Autodesk Fusion 360 part; units mm, degrees
(part 2 of 2)
  constraint perpendicular L102 L652
  constraint perpendicular L102 L126
  constraint perpendicular L121 L652
  constraint perpendicular L117 L121
  constraint perpendicular L572 L652
  constraint perpendicular L47 L572
  constraint perpendicular L83 L132
  constraint perpendicular L185 L219
  constraint perpendicular L70 L132
  constraint perpendicular L55 L185
  constraint perpendicular L132 L662
  constraint perpendicular L185 L660
  constraint perpendicular L132 L188
  constraint perpendicular L183 L185
  constraint perpendicular L16 L132
  constraint perpendicular L185 L686
  constraint perpendicular L132 L681
  constraint perpendicular L185 L684
  constraint perpendicular L132 L676
  constraint perpendicular L185 L690
  constraint perpendicular L685 L690
  constraint perpendicular L685 L689
  constraint perpendicular L690 L695
  constraint perpendicular L693 L695
  constraint perpendicular L690 L691
  constraint perpendicular L691 L703
  constraint perpendicular L690 L694
  constraint perpendicular L679 L694
  constraint perpendicular L683 L690
  constraint perpendicular L682 L683
  constraint perpendicular L146 L682
  constraint coincident L671.start L185
  constraint perpendicular L185 L671
  constraint perpendicular L671 L677
  constraint perpendicular L185 L680
  constraint perpendicular L680 L688
  constraint perpendicular L687 L688
  constraint perpendicular L669 L687
  constraint perpendicular L673 L688
  constraint perpendicular L673 L674
  constraint perpendicular L675 L688
  constraint perpendicular L670 L675
  constraint perpendicular L678 L688
  constraint perpendicular L678 L701
  constraint perpendicular L33 L688
  constraint perpendicular L33 L58
  constraint coincident L82.end L185
  constraint perpendicular L82 L185
  constraint coincident L116.start L185
  constraint perpendicular L116 L134
  constraint perpendicular L100 L650
  constraint perpendicular L134 L278
  constraint perpendicular L650 L667
  constraint perpendicular L134 L647
  constraint perpendicular L104 L647
  constraint perpendicular L134 L657
  constraint perpendicular L136 L647
  constraint perpendicular L134 L659
  constraint perpendicular L89 L659
  constraint coincident L553.start L185
  constraint perpendicular L185 L591
  constraint vertical L558
  constraint perpendicular L123 L558
  constraint perpendicular L123 L642
  constraint perpendicular L642 L653
  constraint perpendicular L653 L666
  constraint perpendicular L658 L666
  constraint perpendicular L645 L653
  constraint perpendicular L101 L645
  constraint perpendicular L275 L653
  constraint perpendicular L153 L275
  constraint perpendicular L106 L653
  constraint perpendicular L124 L558
  constraint coincident L553.end L185
  constraint perpendicular L185 L581
  constraint perpendicular L256 L581
  constraint perpendicular L313 L553
  constraint perpendicular L191 L313
  constraint perpendicular L256 L348
  constraint perpendicular L313 L539
  constraint perpendicular L539 L583
  constraint perpendicular L479 L583
  constraint perpendicular L499 L539
  constraint perpendicular L499 L527
  constraint perpendicular L539 L603
  constraint perpendicular L475 L603
  constraint perpendicular L496 L539
  constraint perpendicular L496 L593
  constraint perpendicular L475 L626
  constraint perpendicular L586 L591
  constraint perpendicular L289 L475
  constraint perpendicular L289 L619
  constraint perpendicular L475 L536
  constraint perpendicular L289 L490
  constraint perpendicular L475 L633
  constraint perpendicular L226 L625
  constraint perpendicular L198 L226
  constraint perpendicular L198 L216
  constraint perpendicular L216 L413
  constraint perpendicular L399 L479
  constraint perpendicular L229 L399
  constraint perpendicular L229 L376
  constraint perpendicular L207 L399
  constraint perpendicular L229 L407
  constraint perpendicular L241 L399
  constraint perpendicular L229 L451
  constraint perpendicular L230 L399
  constraint perpendicular L229 L377
  constraint perpendicular L351 L399
  constraint perpendicular L229 L404
  constraint perpendicular L68 L399
  constraint perpendicular L229 L303
  constraint perpendicular L35 L399
  constraint perpendicular L229 L276
  constraint perpendicular L63 L399
  constraint coincident L400.end L185
  constraint perpendicular L185 L400
  constraint perpendicular L106 L579
  constraint perpendicular L185 L379
  constraint perpendicular L106 L386
  constraint perpendicular L185 L321
  constraint perpendicular L106 L394
  constraint perpendicular L52 L185
  constraint perpendicular L106 L212
  constraint perpendicular L185 L326
  constraint perpendicular L106 L383
  constraint perpendicular L185 L406
  constraint perpendicular L106 L292
  constraint perpendicular L25 L185
  constraint perpendicular L106 L262
  constraint perpendicular L185 L422
  constraint perpendicular L106 L361
  constraint perpendicular L361 L384
  constraint perpendicular L223 L499
  constraint perpendicular L238 L527
  constraint perpendicular L213 L499
  constraint perpendicular L225 L527
  constraint perpendicular L392 L499
  constraint perpendicular L73 L412
  constraint perpendicular L242 L405
  constraint perpendicular L392 L563
  constraint perpendicular L73 L373
  constraint perpendicular L484 L541
  constraint perpendicular L541 L621
  constraint perpendicular L484 L611
  constraint perpendicular L487 L611
  constraint perpendicular L282 L484
  constraint perpendicular L282 L470
  constraint perpendicular L484 L573
  constraint perpendicular L185 L498
  constraint perpendicular L330 L484
  constraint perpendicular L185 L190
  constraint perpendicular L335 L484
  constraint perpendicular L185 L482
  constraint perpendicular L364 L484
  constraint perpendicular L185 L363
  constraint perpendicular L310 L484
  constraint perpendicular L185 L318
  constraint perpendicular L306 L484
  constraint perpendicular L306 L338
  constraint perpendicular L234 L338
  constraint perpendicular L221 L306
  constraint perpendicular L221 L540
  constraint perpendicular L538 L579
  constraint vertical L197
  constraint perpendicular L72 L197
  constraint perpendicular L27 L72
  constraint perpendicular L144 L197
  constraint perpendicular L29 L144
  constraint perpendicular L85 L197
  constraint perpendicular L46 L85
  constraint perpendicular L197 L248
  measures "d65" distance of L40.start L40.end
  measures "d66" distance of L40.end L43.start
  measures "d67" distance of L43.start L28.start
  measures "d68" distance of L28.start L28.end
  measures "d69" distance of L227.end L28.end
  measures "d70" distance of L227.end L75.start
  measures "d71" distance of L75.start L59.start
  measures "d72" distance of L54.start L59.start
  measures "d73" distance of L54.end L67.start
  measures "d74" distance of L67.start L67.end
  measures "d75" distance of L530.end L67.end
  measures "d76" distance of L329.start L562.end
  measures "d77" distance of L409.start L67.end
  measures "d78" distance of L481.start L481.end
  measures "d79" distance of L562.end L567.start
  measures "d80" distance of L567.start L513.start
  measures "d81" distance of L513.start L301.start
  measures "d82" distance of L505.start L481.end
  measures "d83" distance of L296.end L91.start
extrude "Extrude17" add sketch "Sketch10" along normal blind 1 separate body contours L6 L9 L11 L15 L17 L19 L20 L21 L33 L58 L82 L92 L103 L128 L129 L132 L140 L148 L149 L152 L157 L180 L182 L185 L189 L442 L643 L650 L661 L668 L669 L670 L671 L673 L674 L675 L677 L678 L680 L687 L688 L701 L702 | L89 L100 L104 L116 L136 L185 L278 L591 L647 L657 L659 L667 | L35 L63 L68 L185 L191 L198 L207 L216 L226 L229 L230 L241 L256 L276 L289 L303 L313 L348 L351 L376 L377 L399 L400 L404 L407 L413 L451 L475 L479 L490 L496 L499 L527 L536 L539 L581 L583 L586 L593 L603 L619 L625 L626 L633 L644 | L45 L57 L80 L86 L185 L252 L257 L324 L331 L357 L358 L367 L380 L433 L474 L485 L504 L523 L537 L544 L569 L570 L638 | L31 L34 L42 L44 L48 L64 L65 L107 L145 L185 L192 L201 L208 L210 L220 L244 L246 L264 L283 L308 L336 L341 L355 L356 L372 L375 L387 L389 L390 L403 L424 L426 L440 L457 L462 L467 L491 L502 L507 L542 L574 L584 L589 L592 L599 L629 L646 L654 | L93 L108 L122 L156 L171 L178 L179 L445 L452 L644 L696 | L91 L115 L131 L150 L163 L170 L423 L429 L460 L463 L471 L696 | L28 L43 L54 L59 L67 L75 L196 L227 L232 L247 L301 L329 L513 L530 L562 L567 L612 L624 L646 L696 | L114 L154 L166 L172 L259 L290 L296 L421 L431 L432 L436 L456 L468 L511 L532 L534 L550 L551 L600 L615 L622 L696 | L71 L94 L118 L138 L204 L209 L218 L222 L237 L245 L251 L255 L273 L274 L280 L287 L288 L291 L300 L305 L309 L311 L315 L322 L327 L337 L340 L347 L350 L354 L362 L398 L402 L410 L414 L427 L465 L472 L480 L552 L556 L566 L575 L577 L594 L598 L604 L609 L617 L618 L623 L631 L634 L696 | L66 L79 L151 L228 L235 L297 L298 L304 L382 L385 L497 L554 | L95 L267 L269 L469 L533 L547 L560 L639 | L97 L98 L109 L147 L158 L165 L265 L293 L307 L328 L333 L344 L369 L381 L393 L453 L493 L531 L571 L608 L616 L635 | L261 L271 L294 L334 L515 L524 L568 L580 L627 makes body 4 at (-2.3278, 31.3686, -89.3333) makes body 5 at (-2.0859, 30.3983, -78.6667) makes body 6 at (2.9945, 10.0221, -78.6667) makes body 7 at (0.8978, 18.4314, -126) makes body 8 at (2.6719, 11.3159, -75.6667) makes body 9 at (-3.5374, 36.2201, -72) makes body 10 at (-3.9406, 37.8373, -108.6667) makes body 11 at (-5.0696, 42.3653, -92.3333) makes body 12 at (-5.2309, 43.0122, -51) makes body 13 at (3.9622, 6.1409, -82.3333) makes body 14 at (3.6396, 7.4347, -104.3333) makes body 15 at (2.6719, 11.3159, -50.3333) makes body 16 at (-1.844, 29.428, -92.3333) makes body 17 at (-3.6987, 36.867, -128.3333)
scale "Scale1" factor 0.2 about (4.446, 4.2004, -129) bodies 13 17 14 6 15 5 4 10 11 8 12 9 16 7
move_body "Move1" bodies 10 14 8 11 17 13 15 12 16 6 5 9 4 7 to x (1, 0, 0) y (0, 1, 0) z (0, 0, 1) at (1.938, -3.6393, 122)
move_body "Move2" bodies 7 15 9 5 12 6 14 8 13 10 4 11 17 16 to x (1, 0, 0) y (0, 1, 0) z (0, 0, 1) at (0, 0, -0.5)
move_body "Move3" bodies 12 13 6 9 5 4 14 11 17 8 10 16 15 7 to x (1, 0, 0) y (0, 1, 0) z (0, 0, 1) at (4.8515, 1.2096, 0)
extrude "Extrude18" cut 14 faces at (9.9614, 6.8809, -6.5667) (9.8162, 7.4631, -4.3667) (9.8807, 7.2044, 0.4333) (9.413, 9.0803, -0.1667) (9.9775, 6.8162, -0.1667) (9.6388, 8.1747, 3.9) (9.9291, 7.0103, 2.5667) (9.3001, 9.5331, 8.1) (11.0097, 2.6763, 8.2333) (11.1387, 2.1588, 4.6333) (10.9613, 2.8704, 4.0333) (11.1387, 2.1588, 1.8333) (11.0742, 2.4176, -2.5667) (11.3645, 1.2532, -6.9) along direction (-0.970296, -0.241922, 0) blind 7 on bodies 4 5 6 7 8 9 10 11 12 13 14 15 16 17 bodies 2
sketch "Sketch11" plane through (0, 0, 0) normal (0, 0, 1) x (1, 0, 0)
  line L0 (-45, 0) -> (-43, 0)
  line L1 (-43, 0) -> (-43, 10)
  line L2 (-43, 10) -> (-45, 10)
  line L3 (-45, 10) -> (-45, 0)
  line L4 (-45, 0) -> (-47.7, 0)
  line L5 (-47.7, 0) -> (-49.7, 0)
  line L6 (-49.7, 0) -> (-49.7, 3)
  line L7 (-49.7, 3) -> (-47.7, 3)
  line L8 (-47.7, 3) -> (-47.7, 0)
  line L9 (-43, 0) -> (-36.3, 0)
  line L10 (-36.3, 0) -> (-36.3, 19.5)
  line L11 (-36.3, 19.5) -> (-43, 19.5)
  line L12 (-43, 19.5) -> (-43, 0)
  line L13 (-43, 19.5) -> (-41, 19.5)
  line L14 (-41, 19.5) -> (-41, 22.5)
  line L15 (-41, 22.5) -> (-43, 22.5)
  line L16 (-43, 22.5) -> (-43, 19.5)
  line L17 (-36.3, 19.5) -> (-38.3, 19.5)
  line L18 (-38.3, 19.5) -> (-38.3, 29.5)
  line L19 (-38.3, 29.5) -> (-36.3, 29.5)
  line L20 (-36.3, 29.5) -> (-36.3, 19.5)
  line L21 (-36.3, 0) -> (-29.6, 0)
  line L22 (-29.6, 0) -> (-29.6, 39)
  line L23 (-29.6, 39) -> (-36.3, 39)
  line L24 (-36.3, 39) -> (-36.3, 0)
  line L25 (-36.3, 39) -> (-34.3, 39)
  line L26 (-34.3, 39) -> (-34.3, 42)
  line L27 (-34.3, 42) -> (-36.3, 42)
  line L28 (-36.3, 42) -> (-36.3, 39)
  line L29 (-29.6, 39) -> (-31.6, 39)
  line L30 (-31.6, 39) -> (-31.6, 49)
  line L31 (-31.6, 49) -> (-29.6, 49)
  line L32 (-29.6, 49) -> (-29.6, 39)
  line L33 (-29.6, 0) -> (-22.9, 0)
  line L34 (-22.9, 0) -> (-22.9, 58.5)
  line L35 (-22.9, 58.5) -> (-29.6, 58.5)
  line L36 (-29.6, 58.5) -> (-29.6, 0)
  line L37 (-29.6, 58.5) -> (-27.6, 58.5)
  line L38 (-27.6, 58.5) -> (-27.6, 61.5)
  line L39 (-27.6, 61.5) -> (-29.6, 61.5)
  line L40 (-29.6, 61.5) -> (-29.6, 58.5)
  line L41 (-22.9, 58.5) -> (-24.9, 58.5)
  line L42 (-24.9, 58.5) -> (-24.9, 68.5)
  line L43 (-24.9, 68.5) -> (-22.9, 68.5)
  line L44 (-22.9, 68.5) -> (-22.9, 58.5)
  line L45 (-22.9, 0) -> (-49.7, 0)
  line L46 (-49.7, 0) -> (-49.7, -2)
  line L47 (-49.7, -2) -> (-22.9, -2)
  line L48 (-22.9, -2) -> (-22.9, 0)
  line L49 (-49.7, 0) -> (-51.7, 0)
  line L50 (-51.7, 0) -> (-51.7, -2)
  line L51 (-51.7, -2) -> (-49.7, -2)
  line L52 (-49.7, -2) -> (-49.7, 0)
  line L53 (-22.9, 0) -> (-20.9, 0)
  line L54 (-20.9, 0) -> (-20.9, -2)
  line L55 (-20.9, -2) -> (-22.9, -2)
  line L56 (-22.9, -2) -> (-22.9, 0)
  dimension "d89" = 2
  dimension "d90" = 10
  dimension "d91" = 2.7
  dimension "d92" = 2
  dimension "d93" = 3
  dimension "d94" = 19.5
  dimension "d95" = 6.7
  dimension "d96" = 3
  dimension "d97" = 10
  dimension "d98" = 2
  dimension "d99" = 39
  dimension "d100" = 6.7
  dimension "d101" = 2
  dimension "d102" = 3
  dimension "d103" = 10
  dimension "d104" = 2
  dimension "d105" = 58.5
  dimension "d106" = 6.7
  dimension "d107" = 2
  dimension "d108" = 3
  dimension "d109" = 2
  dimension "d110" = 10
  dimension "d111" = 2
  dimension "d112" = 2
  dimension "d113" = 2
  constraint horizontal L0
  constraint vertical L1
  constraint horizontal L2
  constraint vertical L3
  constraint perpendicular L3 L4
  constraint horizontal L5
  constraint vertical L6
  constraint horizontal L7
  constraint vertical L8
  constraint horizontal L9
  constraint vertical L10
  constraint horizontal L11
  constraint vertical L12
  constraint horizontal L13
  constraint vertical L14
  constraint horizontal L15
  constraint vertical L16
  constraint horizontal L17
  constraint vertical L18
  constraint horizontal L19
  constraint vertical L20
  constraint horizontal L21
  constraint vertical L22
  constraint horizontal L23
  constraint vertical L24
  constraint horizontal L25
  constraint vertical L26
  constraint horizontal L27
  constraint vertical L28
  constraint horizontal L29
  constraint vertical L30
  constraint horizontal L31
  constraint vertical L32
  constraint horizontal L33
  constraint vertical L34
  constraint horizontal L35
  constraint vertical L36
  constraint horizontal L37
  constraint vertical L38
  constraint horizontal L39
  constraint vertical L40
  constraint horizontal L41
  constraint vertical L42
  constraint horizontal L43
  constraint vertical L44
  constraint horizontal L45
  constraint vertical L46
  constraint horizontal L47
  constraint vertical L48
  constraint horizontal L49
  constraint vertical L50
  constraint horizontal L51
  constraint vertical L52
  constraint horizontal L53
  constraint vertical L54
  constraint horizontal L55
  constraint vertical L56
  measures "d89" distance of L0.start L0.end
  measures "d90" distance of L0.start L2.end
  measures "d91" distance of L0.start L4.end
  measures "d92" distance of L4.end L5.end
  measures "d93" distance of L4.end L7.end
  measures "d94" distance of L0.end L11.end
  measures "d95" distance of L0.end L9.end
  measures "d96" distance of L11.end L15.end
  measures "d97" distance of L10.end L19.end
  measures "d98" distance of L10.end L17.end
  measures "d99" distance of L9.end L23.end
  measures "d100" distance of L9.end L21.end
  measures "d101" distance of L23.end L25.end
  measures "d102" distance of L23.end L27.end
  measures "d103" distance of L22.end L31.end
  measures "d104" distance of L22.end L29.end
  measures "d105" distance of L21.end L35.end
  measures "d106" distance of L21.end L33.end
  measures "d107" distance of L35.end L37.end
  measures "d108" distance of L35.end L39.end
  measures "d109" distance of L34.end L41.end
  measures "d110" distance of L34.end L43.end
  measures "d111" distance of L33.end L47.end
  measures "d112" distance of L5.end L49.end
  measures "d113" distance of L33.end L53.end
extrude "Extrude19" add sketch "Sketch11" along normal blind 13 and the other way blind 13 separate body makes body 18
chamfer "Chamfer1" distance 12.5 distance2 2 1 edges at (-29.6, 49, 0) measured on face at (-29.6, 57.3333, 4.3333) on bodies 18
chamfer "Chamfer2" distance 12.5 distance2 2 1 edges at (-36.3, 29.5, 0) measured on face at (-36.3, 33.6667, 4.3333) on bodies 18
chamfer "Chamfer3" distance 12.5 distance2 2 1 edges at (-43, 10, 0) measured on face at (-43, 18.3333, -4.3333) on bodies 18
chamfer "Chamfer4" distance 3 distance2 2 1 edges at (-49.7, 0, 0) measured on face at (-49.7, 2, 4.3333) on bodies 18
sketch "Sketch12" plane through (0, 0, 13) normal (0, 0, 1) x (1, 0, 0)
  line L0 (-22.9, 0) -> (-22.9, 68.5)
  line L1 (-22.9, 68.5) -> (-24.9, 68.5)
  line L2 (-24.9, 68.5) -> (-24.9, 58.5)
  line L3 (-24.9, 58.5) -> (-27.6, 58.5)
  line L4 (-27.6, 58.5) -> (-27.6, 61.5)
  line L5 (-27.6, 61.5) -> (-29.6, 61.5)
  line L6 (-29.6, 61.5) -> (-31.6, 49)
  line L7 (-31.6, 49) -> (-31.6, 39)
  line L8 (-31.6, 39) -> (-34.3, 39)
  line L9 (-34.3, 39) -> (-34.3, 42)
  line L10 (-34.3, 42) -> (-36.3, 42)
  line L11 (-36.3, 42) -> (-38.3, 29.5)
  line L12 (-38.3, 29.5) -> (-38.3, 19.5)
  line L13 (-38.3, 19.5) -> (-41, 19.5)
  line L14 (-41, 19.5) -> (-41, 22.5)
  line L15 (-41, 22.5) -> (-43, 22.5)
  line L16 (-43, 22.5) -> (-45, 10)
  line L17 (-45, 10) -> (-45, 0)
  line L18 (-45, 0) -> (-47.7, 0)
  line L19 (-47.7, 0) -> (-47.7, 3)
  line L20 (-47.7, 3) -> (-49.7, 3)
  line L21 (-49.7, 3) -> (-51.7, 0)
  line L22 (-51.7, 0) -> (-51.7, -2)
  line L23 (-51.7, -2) -> (-20.9, -2)
  line L24 (-20.9, -2) -> (-20.9, 0)
  line L25 (-20.9, 0) -> (-22.9, 0)
  line L26 (-51.7, -2) -> (-20.9, -2)
  line L27 (-20.9, -2) -> (-20.9, 0)
  line L28 (-20.9, 0) -> (-51.7, 0)
  line L29 (-51.7, 0) -> (-51.7, -2)
  constraint horizontal L26
  constraint vertical L27
  constraint horizontal L28
  constraint vertical L29
  constraint coincident L24.end L25.start
  constraint coincident L22.end L23.start
extrude "Extrude20" add sketch "Sketch12" along normal blind 4 contours L18 L22 L23 L24 L25 L26 L27 L28 L29 bodies 18
sketch "Sketch13" plane through (0, 0, -13) normal (0, 0, -1) x (-1, 0, 0)
  line L0 (22.9, 68.5) -> (22.9, 0)
  line L1 (22.9, 0) -> (20.9, 0)
  line L2 (20.9, 0) -> (20.9, -2)
  line L3 (20.9, -2) -> (51.7, -2)
  line L4 (51.7, -2) -> (51.7, 0)
  line L5 (51.7, 0) -> (49.7, 3)
  line L6 (49.7, 3) -> (47.7, 3)
  line L7 (47.7, 3) -> (47.7, 0)
  line L8 (47.7, 0) -> (45, 0)
  line L9 (45, 0) -> (45, 10)
  line L10 (45, 10) -> (43, 22.5)
  line L11 (43, 22.5) -> (41, 22.5)
  line L12 (41, 22.5) -> (41, 19.5)
  line L13 (41, 19.5) -> (38.3, 19.5)
  line L14 (38.3, 19.5) -> (38.3, 29.5)
  line L15 (38.3, 29.5) -> (36.3, 42)
  line L16 (36.3, 42) -> (34.3, 42)
  line L17 (34.3, 42) -> (34.3, 39)
  line L18 (34.3, 39) -> (31.6, 39)
  line L19 (31.6, 39) -> (31.6, 49)
  line L20 (31.6, 49) -> (29.6, 61.5)
  line L21 (29.6, 61.5) -> (27.6, 61.5)
  line L22 (27.6, 61.5) -> (27.6, 58.5)
  line L23 (27.6, 58.5) -> (24.9, 58.5)
  line L24 (24.9, 58.5) -> (24.9, 68.5)
  line L25 (24.9, 68.5) -> (22.9, 68.5)
  line L26 (20.9, -2) -> (51.7, -2)
  line L27 (51.7, -2) -> (51.7, 0)
  line L28 (51.7, 0) -> (20.9, 0)
  line L29 (20.9, 0) -> (20.9, -2)
  constraint horizontal L26
  constraint vertical L27
  constraint horizontal L28
  constraint vertical L29
  constraint coincident L4.end L5.start
  constraint coincident L2.end L3.start
extrude "Extrude21" add sketch "Sketch13" along normal blind 2 contours L1 L2 L3 L4 L8 L26 L27 L28 L29 bodies 18
extrude "Extrude22" cut 1 faces at (-31.1667, -1.3333, 17) along direction (0, 0, -1) blind 2 on bodies 18 bodies 18
sketch "Sketch14" plane through (0, 0, 13) normal (0, 0, 1) x (1, 0, 0)
  line L0 (-45, 0) -> (-22.9, 0)
  line L1 (-22.9, 0) -> (-22.9, 68.5)
  line L2 (-22.9, 68.5) -> (-24.9, 68.5)
  line L3 (-24.9, 68.5) -> (-24.9, 58.5)
  line L4 (-24.9, 58.5) -> (-27.6, 58.5)
  line L5 (-27.6, 58.5) -> (-27.6, 61.5)
  line L6 (-27.6, 61.5) -> (-29.6, 61.5)
  line L7 (-29.6, 61.5) -> (-31.6, 49)
  line L8 (-31.6, 49) -> (-31.6, 39)
  line L9 (-31.6, 39) -> (-34.3, 39)
  line L10 (-34.3, 39) -> (-34.3, 42)
  line L11 (-34.3, 42) -> (-36.3, 42)
  line L12 (-36.3, 42) -> (-38.3, 29.5)
  line L13 (-38.3, 29.5) -> (-38.3, 19.5)
  line L14 (-38.3, 19.5) -> (-41, 19.5)
  line L15 (-41, 19.5) -> (-41, 22.5)
  line L16 (-41, 22.5) -> (-43, 22.5)
  line L17 (-43, 22.5) -> (-45, 10)
  line L18 (-45, 10) -> (-45, 0)
  line L19 (-43, 22.5) -> (-41, 22.5)
  line L20 (-41, 22.5) -> (-41, 0)
  line L21 (-41, 0) -> (-43, 0)
  line L22 (-43, 0) -> (-43, 22.5)
  line L23 (-41, 19.5) -> (-38.3, 19.5)
  line L24 (-38.3, 19.5) -> (-38.3, 0)
  line L25 (-38.3, 0) -> (-41, 0)
  line L26 (-41, 0) -> (-41, 19.5)
  line L27 (-38.3, 19.5) -> (-22.9, 19.5)
  line L28 (-22.9, 19.5) -> (-22.9, 0)
  line L29 (-22.9, 0) -> (-38.3, 0)
  line L30 (-38.3, 0) -> (-38.3, 19.5)
  constraint horizontal L19
  constraint vertical L20
  constraint horizontal L21
  constraint vertical L22
  constraint coincident L0 L20.end
  constraint coincident L16.end L17.start
  constraint horizontal L23
  constraint vertical L24
  constraint horizontal L25
  constraint vertical L26
  constraint coincident L0 L24.end
  constraint coincident L14.end L15.start
  constraint horizontal L27
  constraint vertical L28
  constraint horizontal L29
  constraint vertical L30
  constraint coincident L0.end L1.start
extrude "Extrude23" add sketch "Sketch14" along normal blind 2 contours L0 L15 L16 L19 L20 L21 L22 L26 | L0 L14 L20 L23 L24 L25 L26 L30 | L0 L1 L24 L27 L28 L29 L30 bodies 18
sketch "Sketch15" plane through (0, 0, 13) normal (0, 0, 1) x (1, 0, 0)
  line L0 (-38.3, 19.5) -> (-22.9, 19.5)
  line L1 (-22.9, 19.5) -> (-22.9, 68.5)
  line L2 (-22.9, 68.5) -> (-24.9, 68.5)
  line L3 (-24.9, 68.5) -> (-24.9, 58.5)
  line L4 (-24.9, 58.5) -> (-27.6, 58.5)
  line L5 (-27.6, 58.5) -> (-27.6, 61.5)
  line L6 (-27.6, 61.5) -> (-29.6, 61.5)
  line L7 (-29.6, 61.5) -> (-31.6, 49)
  line L8 (-31.6, 49) -> (-31.6, 39)
  line L9 (-31.6, 39) -> (-34.3, 39)
  line L10 (-34.3, 39) -> (-34.3, 42)
  line L11 (-34.3, 42) -> (-36.3, 42)
  line L12 (-36.3, 42) -> (-38.3, 29.5)
  line L13 (-38.3, 29.5) -> (-38.3, 19.5)
  line L14 (-36.3, 42) -> (-34.3, 42)
  line L15 (-34.3, 42) -> (-34.3, 19.5)
  line L16 (-34.3, 19.5) -> (-36.3, 19.5)
  line L17 (-36.3, 19.5) -> (-36.3, 42)
  line L18 (-34.3, 39) -> (-22.9, 39)
  line L19 (-22.9, 39) -> (-22.9, 19.5)
  line L20 (-22.9, 19.5) -> (-34.3, 19.5)
  line L21 (-34.3, 19.5) -> (-34.3, 39)
  constraint horizontal L14
  constraint vertical L15
  constraint horizontal L16
  constraint vertical L17
  constraint coincident L0 L15.end
  constraint coincident L11.end L12.start
  constraint horizontal L18
  constraint vertical L19
  constraint horizontal L20
  constraint vertical L21
  constraint coincident L0.end L1.start
  constraint coincident L9.end L10.start
extrude "Extrude24" add sketch "Sketch15" along normal blind 2 contours L0 L10 L11 L14 L15 L16 L17 L21 | L0 L1 L9 L15 L18 L19 L20 L21 bodies 18
sketch "Sketch16" plane through (0, 0, 13) normal (0, 0, 1) x (1, 0, 0)
  line L0 (-31.6, 39) -> (-22.9, 39)
  line L1 (-22.9, 39) -> (-22.9, 68.5)
  line L2 (-22.9, 68.5) -> (-24.9, 68.5)
  line L3 (-24.9, 68.5) -> (-24.9, 58.5)
  line L4 (-24.9, 58.5) -> (-27.6, 58.5)
  line L5 (-27.6, 58.5) -> (-27.6, 61.5)
  line L6 (-27.6, 61.5) -> (-29.6, 61.5)
  line L7 (-29.6, 61.5) -> (-31.6, 49)
  line L8 (-31.6, 49) -> (-31.6, 39)
  line L9 (-29.6, 61.5) -> (-27.6, 61.5)
  line L10 (-27.6, 61.5) -> (-27.6, 39)
  line L11 (-27.6, 39) -> (-29.6, 39)
  line L12 (-29.6, 39) -> (-29.6, 61.5)
  line L13 (-27.6, 39) -> (-22.9, 39)
  line L14 (-22.9, 39) -> (-22.9, 58.5)
  line L15 (-22.9, 58.5) -> (-27.6, 58.5)
  line L16 (-27.6, 58.5) -> (-27.6, 39)
  constraint horizontal L9
  constraint vertical L10
  constraint horizontal L11
  constraint vertical L12
  constraint coincident L0 L10.end
  constraint coincident L6.end L7.start
  constraint horizontal L13
  constraint vertical L14
  constraint horizontal L15
  constraint vertical L16
  constraint coincident L1 L14.end
extrude "Extrude25" add sketch "Sketch16" along normal blind 2 contours L0 L5 L6 L9 L10 L11 L12 L16 | L0 L1 L4 L10 L13 L14 L15 L16 bodies 18
sketch "Sketch17" plane through (0, 0, -13) normal (0, 0, -1) x (-1, 0, 0)
  line L0 (22.9, 0) -> (45, 0)
  line L1 (45, 0) -> (45, 10)
  line L2 (45, 10) -> (43, 22.5)
  line L3 (43, 22.5) -> (41, 22.5)
  line L4 (41, 22.5) -> (41, 19.5)
  line L5 (41, 19.5) -> (38.3, 19.5)
  line L6 (38.3, 19.5) -> (38.3, 29.5)
  line L7 (38.3, 29.5) -> (36.3, 42)
  line L8 (36.3, 42) -> (34.3, 42)
  line L9 (34.3, 42) -> (34.3, 39)
  line L10 (34.3, 39) -> (31.6, 39)
  line L11 (31.6, 39) -> (31.6, 49)
  line L12 (31.6, 49) -> (29.6, 61.5)
  line L13 (29.6, 61.5) -> (27.6, 61.5)
  line L14 (27.6, 61.5) -> (27.6, 58.5)
  line L15 (27.6, 58.5) -> (24.9, 58.5)
  line L16 (24.9, 58.5) -> (24.9, 68.5)
  line L17 (24.9, 68.5) -> (22.9, 68.5)
  line L18 (22.9, 68.5) -> (22.9, 0)
  line L19 (43, 22.5) -> (41, 22.5)
  line L20 (41, 22.5) -> (41, 0)
  line L21 (41, 0) -> (43, 0)
  line L22 (43, 0) -> (43, 22.5)
  line L23 (41, 19.5) -> (22.9, 19.5)
  line L24 (22.9, 19.5) -> (22.9, 0)
  line L25 (22.9, 0) -> (41, 0)
  line L26 (41, 0) -> (41, 19.5)
  line L27 (34.3, 42) -> (36.3, 42)
  line L28 (36.3, 42) -> (36.3, 19.5)
  line L29 (36.3, 19.5) -> (34.3, 19.5)
  line L30 (34.3, 19.5) -> (34.3, 42)
  line L31 (34.3, 39) -> (22.9, 39)
  line L32 (22.9, 39) -> (22.9, 19.5)
  line L33 (22.9, 19.5) -> (34.3, 19.5)
  line L34 (34.3, 19.5) -> (34.3, 39)
  line L35 (27.6, 61.5) -> (29.6, 61.5)
  line L36 (29.6, 61.5) -> (29.6, 39)
  line L37 (29.6, 39) -> (27.6, 39)
  line L38 (27.6, 39) -> (27.6, 61.5)
  line L39 (27.6, 58.5) -> (22.9, 58.5)
  line L40 (22.9, 58.5) -> (22.9, 39)
  line L41 (22.9, 39) -> (27.6, 39)
  line L42 (27.6, 39) -> (27.6, 58.5)
  dimension "d138" = 2
  constraint horizontal L19
  constraint vertical L20
  constraint horizontal L21
  constraint vertical L22
  constraint coincident L0 L20.end
  constraint coincident L2.end L3.start
  constraint horizontal L23
  constraint vertical L24
  constraint horizontal L25
  constraint vertical L26
  constraint coincident L0.start L18.end
  constraint coincident L4.end L5.start
  constraint horizontal L27
  constraint vertical L28
  constraint horizontal L29
  constraint vertical L30
  constraint coincident L23 L28.end
  constraint coincident L8.end L9.start
  constraint horizontal L31
  constraint vertical L32
  constraint horizontal L33
  constraint vertical L34
  constraint coincident L9.end L10.start
  constraint horizontal L35
  constraint vertical L36
  constraint horizontal L37
  constraint vertical L38
  constraint coincident L13.end L14.start
  constraint horizontal L39
  constraint vertical L40
  constraint horizontal L41
  constraint vertical L42
  constraint coincident L14.end L15.start
  measures "d138" distance of L13.end L12.end
extrude "Extrude26" add sketch "Sketch17" along normal blind 2 contours L0 L5 L18 L20 L23 L24 L25 L26 L29 L33 | L0 L3 L4 L19 L20 L21 L22 L26 | L10 L18 L23 L30 L31 L32 L33 L34 L37 L41 | L15 L18 L31 L38 L39 L40 L41 L42 | L8 L9 L23 L27 L28 L29 L30 L34 | L13 L14 L31 L35 L36 L37 L38 L42 bodies 18
sketch "Sketch18" plane through (0, 0, -15) normal (0, 0, -1) x (-1, 0, 0)
  line L0 (20.9, 0) -> (20.9, -2)
  line L1 (20.9, -2) -> (51.7, -2)
  line L2 (51.7, -2) -> (51.7, 0)
  line L3 (51.7, 0) -> (43, 0)
  line L4 (43, 0) -> (43, 22.5)
  line L5 (43, 22.5) -> (41, 22.5)
  line L6 (41, 22.5) -> (41, 19.5)
  line L7 (41, 19.5) -> (36.3, 19.5)
  line L8 (36.3, 19.5) -> (36.3, 42)
  line L9 (36.3, 42) -> (34.3, 42)
  line L10 (34.3, 42) -> (34.3, 39)
  line L11 (34.3, 39) -> (29.6, 39)
  line L12 (29.6, 39) -> (29.6, 61.5)
  line L13 (29.6, 61.5) -> (27.6, 61.5)
  line L14 (27.6, 61.5) -> (27.6, 58.5)
  line L15 (27.6, 58.5) -> (22.9, 58.5)
  line L16 (22.9, 58.5) -> (22.9, 0)
  line L17 (22.9, 0) -> (20.9, 0)
  line L18 (20.9, 0) -> (51.7, 0)
  line L19 (51.7, 0) -> (51.7, -2)
  line L20 (51.7, -2) -> (20.9, -2)
  line L21 (20.9, -2) -> (20.9, 0)
  constraint horizontal L18
  constraint vertical L19
  constraint horizontal L20
  constraint vertical L21
  constraint coincident L1.end L2.start
  constraint coincident L0.start L17.end
extrude "Extrude27" add sketch "Sketch18" along normal blind 2 contours L0 L1 L2 L3 L17 L18 L19 L20 L21 bodies 18
sketch "Sketch19" plane through (0, 0, 15) normal (0, 0, 1) x (1, 0, 0)
  line L0 (-51.7, 0) -> (-51.7, -2)
  line L1 (-51.7, -2) -> (-20.9, -2)
  line L2 (-20.9, -2) -> (-20.9, 0)
  line L3 (-20.9, 0) -> (-22.9, 0)
  line L4 (-22.9, 0) -> (-22.9, 58.5)
  line L5 (-22.9, 58.5) -> (-27.6, 58.5)
  line L6 (-27.6, 58.5) -> (-27.6, 61.5)
  line L7 (-27.6, 61.5) -> (-29.6, 61.5)
  line L8 (-29.6, 61.5) -> (-29.6, 39)
  line L9 (-29.6, 39) -> (-34.3, 39)
  line L10 (-34.3, 39) -> (-34.3, 42)
  line L11 (-34.3, 42) -> (-36.3, 42)
  line L12 (-36.3, 42) -> (-36.3, 19.5)
  line L13 (-36.3, 19.5) -> (-41, 19.5)
  line L14 (-41, 19.5) -> (-41, 22.5)
  line L15 (-41, 22.5) -> (-43, 22.5)
  line L16 (-43, 22.5) -> (-43, 0)
  line L17 (-43, 0) -> (-51.7, 0)
  line L18 (-51.7, 0) -> (-20.9, 0)
  line L19 (-20.9, 0) -> (-20.9, -2)
  line L20 (-20.9, -2) -> (-51.7, -2)
  line L21 (-51.7, -2) -> (-51.7, 0)
  constraint horizontal L18
  constraint vertical L19
  constraint horizontal L20
  constraint vertical L21
  constraint coincident L1.end L2.start
  constraint coincident L0.start L17.end
extrude "Extrude28" add sketch "Sketch19" along normal blind 2 contours L0 L1 L2 L3 L17 L18 L19 L20 L21 bodies 18
draft "Draft11" angle 45 neutral plane through (-43, 0, 15) pull (0, 1, 0) 1 faces at (-41.4333, -1.3333, 17) on bodies 18
draft "Draft12" angle 45 neutral plane through (-43, 0, 15) pull (0, 1, 0) 1 faces at (-31.1667, -0.6667, -17) on bodies 18
draft "Draft13" angle 3.75 neutral plane through (-22.9, 58.5, 13) pull (0, 1, 0) 1 faces at (-34.0667, 6.5, -15) on bodies 18
draft "Draft14" angle 3.75 neutral plane through (-22.9, 58.5, 13) pull (0, 1, 0) 1 faces at (-34.0667, 6.5, 15) on bodies 18
chamfer "Chamfer5" distance 3 distance2 4.36 1 edges at (-42, 22.5, 17.3596) measured on face at (-34.0667, 2.0062, 18.7028) on bodies 18
chamfer "Chamfer6" distance 3 distance2 4.36 1 edges at (-42, 22.5, -17.3596) measured on face at (-34.0667, 2.0062, -18.7028) on bodies 18
chamfer "Chamfer7" distance 3 distance2 3 1 edges at (-35.3, 42, -16.0815) measured on face at (-34.0667, 2.0062, -18.7028) on bodies 18
chamfer "Chamfer8" distance 3 distance2 3 1 edges at (-35.3, 42, 16.0815) measured on face at (-34.0667, 2.0062, 18.7028) on bodies 18
extrude "Extrude29" cut 1 faces at (-20.9, -1.3333, -5.6667) along direction (-1, 0, 0) blind 2 on bodies 18 bodies 18
draft "Draft15" angle 2 neutral plane through (-24.9, 68.5, 0) pull (0, 1, 0) 1 faces at (-22.9, 11.6914, -1.0315) on bodies 18
draft "Draft16" angle 45 neutral plane through (-43, 0, 15) pull (0, 1, 0) 1 faces at (-51.7, -1.3333, -5.6667) on bodies 18
move_body "Move4" bodies 15 14 17 16 6 9 11 8 7 4 5 13 10 12 to x (0.970296, -0.241922, 0) y (0.241922, 0.970296, 0) z (0, 0, 1) at (-1.404, 2.6345, 0)
move_body "Move5" bodies 5 4 7 15 9 6 13 14 11 8 10 17 16 12 to x (1, 0, 0) y (0, 1, 0) z (0, 0, 1) at (0, 32, 0)
move_body "Move6" bodies 7 5 14 11 9 12 6 8 4 17 16 15 10 13 to x (0.999391, 0.034899, 0) y (-0.034899, 0.999391, 0) z (0, 0, 1) at (1.33, -0.3268, 0)
move_body "Move7" bodies 7 9 12 5 6 4 16 8 10 17 14 11 15 13 to x (1, 0, 0) y (0, 1, 0) z (0, 0, 1) at (-25.5, -30, 0)
extrude "Extrude30" cut 14 faces at (-15.7029, 11.6288, 8.1) (-15.6541, 10.2296, 3.9) (-15.6052, 8.8305, 2.5667) (-15.6052, 8.8305, -0.1667) (-15.6192, 9.2302, 0.4333) (-15.6657, 10.5627, -3.4333) (-15.6587, 10.3629, -7.3667) (-15.4051, 3.1006, -6.9) (-15.447, 4.2999, -2.5667) (-15.6983, 11.4955, -0.1667) (-15.4377, 4.0334, 1.8333) (-15.4377, 4.0334, 4.6333) (-15.4563, 4.5664, 8.2333) (-15.4633, 4.7663, 3.1667) along direction (-0.999391, -0.034899, 0) blind 6.208 on bodies 4 5 6 7 8 9 10 11 12 13 14 15 16 17 bodies 18
sketch "Sketch20" plane through (0, 0, 13) normal (0, 0, 1) x (1, 0, 0)
  line L0 (-43, 22.4997) -> (-43, 22.4997)
  line L1 (-43, 22.4997) -> (-45, 10)
  line L2 (-45, 10) -> (-45, 0)
  line L3 (-45, 0) -> (-43, 0)
  line L4 (-43, 0) -> (-43, 22.4997)
  line L5 (-45, 10) -> (-43, 10)
  line L6 (-43, 10) -> (-43, 0)
  line L7 (-43, 0) -> (-45, 0)
  line L8 (-45, 0) -> (-45, 10)
  constraint horizontal L5
  constraint vertical L6
  constraint horizontal L7
  constraint vertical L8
  constraint coincident L3.end L4.start
  constraint coincident L1.end L2.start
extrude "Extrude31" cut sketch "Sketch20" against normal blind 44 contours L1 L4 L5 bodies 18
sketch "Sketch21" plane through (0, 0, 13) normal (0, 0, 1) x (1, 0, 0)
  line L0 (-36.3, 19.5) -> (-36.3, 42)
  line L1 (-36.3, 42) -> (-38.3, 29.5)
  line L2 (-38.3, 29.5) -> (-38.3, 19.5)
  line L3 (-38.3, 19.5) -> (-36.3, 19.5)
  line L4 (-38.3, 29.5) -> (-36.3, 29.5)
  line L5 (-36.3, 29.5) -> (-36.3, 19.5)
  line L6 (-36.3, 19.5) -> (-38.3, 19.5)
  line L7 (-38.3, 19.5) -> (-38.3, 29.5)
  constraint horizontal L4
  constraint vertical L5
  constraint horizontal L6
  constraint vertical L7
  constraint coincident L0.start L3.end
  constraint coincident L1.end L2.start
extrude "Extrude32" cut sketch "Sketch21" against normal blind 35 contours L0 L1 L4 bodies 18
sketch "Sketch22" plane through (0, 0, 13) normal (0, 0, 1) x (1, 0, 0)
  line L0 (-29.6, 39) -> (-29.6, 61.5)
  line L1 (-29.6, 61.5) -> (-31.6, 49)
  line L2 (-31.6, 49) -> (-31.6, 39)
  line L3 (-31.6, 39) -> (-29.6, 39)
  line L4 (-31.6, 49) -> (-29.6, 49)
  line L5 (-29.6, 49) -> (-29.6, 39)
  line L6 (-29.6, 39) -> (-31.6, 39)
  line L7 (-31.6, 39) -> (-31.6, 49)
  constraint horizontal L4
  constraint vertical L5
  constraint horizontal L6
  constraint vertical L7
  constraint coincident L0.start L3.end
  constraint coincident L1.end L2.start
extrude "Extrude33" cut sketch "Sketch22" against normal blind 34 contours L0 L1 L4 bodies 18
chamfer "Chamfer9" distance 3 distance2 3 1 edges at (-28.6, 61.5, -14.8034) measured on face at (-33.2465, 2.0062, -18.7028) on bodies 18
chamfer "Chamfer10" distance 3 distance2 3 1 edges at (-28.6, 61.5, 14.8034) measured on face at (-33.2465, 2.0062, 18.7028) on bodies 18
move_body "Move8" bodies 18 to x (1, 0, 0) y (0, 1, 0) z (0, 0, 1) at (45, 0, 45)
move_face "OffsetFaces1" offset 0.15 1 faces at (0.05, 3.3333, -4.3333) on bodies 2
extrude "Extrude34" cut 14 faces at (5.1073, 1.5482, 6.1) (5.1395, 1.4188, 3.6333) (5.2363, 1.0307, 4.3667) (5.3169, 0.7073, -1.5) (4.1073, 5.5588, 3.1667) (3.8493, 6.5938, 4.5) (3.688, 7.2406, 6.5) (4.1396, 5.4294, -0.4333) (4.3976, 4.3944, -0.3) (3.5751, 7.6934, -0.4333) (3.7202, 7.1112, -4.0333) (3.3332, 8.6637, -6.9) (4.7847, 2.8419, -7.5) (5.1395, 1.4188, -2.8333) along direction (-0.970296, -0.241922, 0) blind 1 on bodies 2 bodies 2
